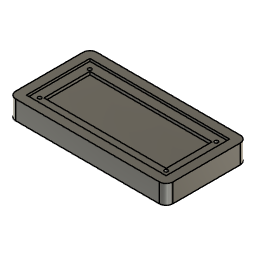
PCB Holder (Autodesk Fusion 360 design; units mm, degrees)
Autodesk Fusion 360 part; units mm, degrees
sketch "Sketch1" plane through (0, 0, 0) normal (0, 0, 1) x (1, 0, 0)
  line L0 (0, 0) -> (103.5, 0)
  line L1 (103.5, 0) -> (103.5, 47)
  line L2 (103.5, 47) -> (0, 47)
  line L3 (0, 47) -> (0, 0)
  line L4 (-6.5, -6.5) -> (110, -6.5)
  line L5 (110, -6.5) -> (110, 53.5)
  line L6 (110, 53.5) -> (-6.5, 53.5)
  line L7 (-6.5, 53.5) -> (-6.5, -6.5)
  line L8 (0, 0) -> (7.051, 0) construction
  circle A0 centre (4.8, 5) radius 1.3
  circle A1 centre (5, 41.9) radius 1.3
  circle A2 centre (98.5, 42.2) radius 1.3
  circle A3 centre (98.5, 5) radius 1.3
  circle A4 centre (-0.5, -0.5) radius 4.25
  circle A5 centre (104, -0.5) radius 4.25
  circle A6 centre (-0.5, 47.5) radius 4.25
  circle A7 centre (104, 47.5) radius 4.25
  line L9 (6.5, 6.5) -> (97, 6.5)
  line L10 (97, 6.5) -> (97, 40.5)
  line L11 (97, 40.5) -> (6.5, 40.5)
  line L12 (6.5, 40.5) -> (6.5, 6.5)
  dimension "d1" = 103.5
  dimension "d2" = 47
  dimension "d3" = 6.5
  dimension "d6" = 2.6
  dimension "d7" = 2.6
  dimension "d9" = 2.6
  dimension "d11" = 2.6
  dimension "d20" = 5
  dimension "d21" = 5.1
  dimension "d22" = 5
  dimension "d23" = 4.8
  dimension "d24" = 5
  dimension "d25" = 5
  dimension "d26" = 4.8
  dimension "d27" = 5
  dimension "d30" = 8.5
  dimension "d31" = 8.5
  dimension "d32" = 8.5
  dimension "d33" = 8.5
  dimension "d34" = 6
  dimension "d36" = 6
  dimension "d37" = 6
  dimension "d38" = 6
  dimension "d39" = 6
  dimension "d40" = 6
  dimension "d41" = 6
  dimension "d42" = 6
  dimension "d45" = -6.5
  constraint horizontal L0
  constraint vertical L1
  constraint horizontal L2
  constraint vertical L3
  constraint coincident L0.start L3.end
  constraint horizontal L8
  measures "d1" distance of L0.start L0.end
  measures "d2" distance of L0.start L2.end
  measures "d6" diameter of A0
  measures "d7" diameter of A1
  measures "d9" diameter of A2
  measures "d11" diameter of A3
  measures "d20" distance of L0 A0.centre
  measures "d21" distance of L2 A1.centre
  measures "d22" distance of L3 A1.centre
  measures "d23" distance of L3 A0.centre
  measures "d24" distance of L1 A2.centre
  measures "d25" distance of L1 A3.centre
  measures "d26" distance of L2 A2.centre
  measures "d27" distance of L0 A3.centre
  measures "d30" diameter of A4
  measures "d31" diameter of A5
  measures "d32" diameter of A6
  measures "d33" diameter of A7
  measures "d34" distance of L6 A6.centre
  measures "d36" distance of L7 A6.centre
  measures "d37" distance of L5 A7.centre
  measures "d38" distance of L6 A7.centre
  measures "d39" distance of L4 A5.centre
  measures "d40" distance of L5 A5.centre
  measures "d41" distance of L4 A4.centre
  measures "d42" distance of L7 A4.centre
extrude "Extrude1" add sketch "Sketch1" along normal blind 10 contours L0 L3 A4 | L0 L3 A4 | L0 L1 L2 L3 A4 A5 A6 A7 | L0 L1 A5 | L0 L1 A5 | L2 L3 A6 | L2 L3 A6 | L1 L2 A7 | L1 L2 A7 | L4 L5 L6 L7 | L9 L10 L11 L12
extrude "Extrude2" add sketch "Sketch1" along normal blind 14 contours L0 L3 A4 | L0 L1 A5 | L2 L3 A6 | L1 L2 A7 | L4 L5 L6 L7 picked at (-2.4457, -2.2102) picked at (105.7715, -2.3893) picked at (-2.4457, 49.2102) picked at (105.7715, 49.3893)
extrude "Extrusion4" add sketch "Sketch1" along normal blind 12.2 contours L0 L3 A4 | L0 L1 L2 L3 A4 A5 A6 A7 | L0 L1 A5 | L2 L3 A6 | L1 L2 A7 picked at (1.6646, 1.6646) picked at (101.8354, 1.6646) picked at (1.6646, 45.3354) picked at (101.8354, 45.3354)
fillet "Fillet1" radius 5 4 edges at (-6.5, 53.5, 7) (110, 53.5, 7) (110, -6.5, 7) (-6.5, -6.5, 7)
extrude "Extrusion3" cut sketch "Sketch1" along normal blind 3.2 contours L0 L3 A4 | L0 L3 A4 | L0 L1 A5 | L0 L1 A5 | L2 L3 A6 | L2 L3 A6 | L1 L2 A7 | L1 L2 A7
